Autodesk Fusion 360 part; units mm, degrees
(part 12 of 13)
  line L9839 (147.471, -118.112) -> (150.319, -115.264)
  line L9840 (149.69, -95.2494) -> (149.801, -95.1926)
  line L9841 (150.319, -98.5784) -> (149.809, -98.0678)
  line L9842 (149.787, -98.039) -> (149.781, -98.0089)
  line L9843 (149.525, -95.573) -> (149.544, -95.4494)
  line L9844 (139.992, -121.691) -> (139.992, -121.713)
  line L9845 (149.544, -95.6966) -> (149.525, -95.573)
  line L9846 (140.035, -118.135) -> (140.038, -118.132)
  line L9847 (137.265, -122.205) -> (137.136, -122.328)
  line L9848 (151.272, -97.8621) -> (151.28, -97.8916)
  line L9849 (151.002, -97.4818) -> (150.975, -97.5348)
  line L9850 (149.772, -95.9386) -> (149.69, -95.8966)
  line L9851 (149.801, -95.1926) -> (149.925, -95.173)
  line L9852 (151.022, -97.3582) -> (151.002, -97.4818)
  line L9853 (149.69, -95.8966) -> (149.601, -95.8081)
  line L9854 (151.265, -97.832) -> (151.272, -97.8621)
  line L9855 (149.792, -98.0469) -> (149.791, -98.0442)
  line L9856 (147.84, -118.96) -> (147.822, -118.974)
  line L9857 (147.752, -118.997) -> (142.062, -118.997)
  line L9858 (151.261, -97.8268) -> (151.265, -97.832)
  line L9859 (149.772, -97.9794) -> (149.772, -95.9387)
  line L9860 (149.781, -98.0089) -> (149.772, -97.9794)
  line L9861 (151.278, -115.495) -> (151.276, -115.498)
  line L9862 (140.017, -118.149) -> (140.035, -118.135)
  line L9863 (139.375, -120.912) -> (139.543, -120.972)
  line L9864 (139.967, -121.89) -> (139.904, -122.056)
  line L9865 (151.244, -115.557) -> (147.84, -118.96)
  line L9866 (139.353, -122.474) -> (139.175, -122.49)
  line L9867 (139.992, -121.713) -> (139.967, -121.89)
  line L9868 (150.387, -97.6818) -> (150.298, -97.5933)
  line L9869 (150.622, -97.7582) -> (150.498, -97.7386)
  line L9870 (138.409, -121.857) -> (138.392, -121.679)
  line L9871 (151.275, -115.504) -> (151.259, -115.53)
  line L9872 (147.817, -118.978) -> (147.811, -118.982)
  line L9873 (142.011, -118.747) -> (147.7, -118.747)
  line L9874 (138.466, -122.026) -> (138.409, -121.857)
  line L9875 (138.682, -122.307) -> (138.558, -122.179)
  line L9876 (150.746, -97.7386) -> (150.622, -97.7582)
  line L9877 (141.981, -118.756) -> (142.011, -118.747)
  line L9878 (138.414, -121.502) -> (138.475, -121.335)
  line L9879 (147.7, -118.747) -> (151.03, -115.417)
  line L9880 (147.811, -118.982) -> (147.781, -118.988)
  line L9881 (139.676, -122.328) -> (139.522, -122.419)
  line L9882 (150.242, -97.2346) -> (150.298, -97.1231)
  line L9883 (139.904, -122.056) -> (139.805, -122.205)
  line L9884 (151.276, -115.498) -> (151.275, -115.504)
  line L9885 (147.822, -118.974) -> (147.819, -118.977)
  line L9886 (147.781, -118.988) -> (147.752, -118.997)
  line L9887 (151.28, -97.8916) -> (151.28, -115.468)
  line L9888 (138.831, -122.405) -> (138.682, -122.307)
  line L9889 (147.819, -118.977) -> (147.817, -118.978)
  line L9890 (138.475, -121.335) -> (138.572, -121.185)
  line L9891 (139.913, -121.345) -> (139.972, -121.513)
  line L9892 (141.946, -118.766) -> (141.951, -118.762)
  line L9893 (150.799, -97.7116) -> (150.746, -97.7386)
  line L9894 (138.998, -122.467) -> (138.831, -122.405)
  line L9895 (139.543, -120.972) -> (139.66, -121.046)
  line L9896 (141.922, -118.784) -> (141.94, -118.77)
  line L9897 (151.28, -115.468) -> (151.277, -115.49)
  line L9898 (138.572, -121.185) -> (138.699, -121.06)
  line L9899 (139.522, -122.419) -> (139.353, -122.474)
  line L9900 (139.805, -122.205) -> (139.676, -122.328)
  line L9901 (139.175, -122.49) -> (138.998, -122.467)
  line L9902 (150.298, -97.5933) -> (150.242, -97.4818)
  line L9903 (141.94, -118.77) -> (141.943, -118.767)
  line L9904 (141.943, -118.767) -> (141.946, -118.766)
  line L9905 (150.242, -97.4818) -> (150.222, -97.3582)
  line L9906 (139.02, -120.909) -> (139.198, -120.891)
  line L9907 (150.498, -97.7386) -> (150.387, -97.6818)
  line L9908 (138.558, -122.179) -> (138.466, -122.026)
  line L9909 (151.03, -97.9434) -> (150.799, -97.7116)
  line L9910 (150.222, -97.3582) -> (150.242, -97.2346)
  line L9911 (118.089, -121.857) -> (118.072, -121.679)
  line L9912 (140.954, -121.502) -> (141.015, -121.335)
  line L9913 (119.356, -122.328) -> (119.202, -122.419)
  line L9914 (119.499, -121.194) -> (119.593, -121.345)
  line L9915 (138.392, -121.679) -> (138.414, -121.502)
  line L9916 (141.015, -121.335) -> (141.112, -121.185)
  line L9917 (142.512, -121.513) -> (142.532, -121.691)
  line L9918 (141.893, -122.474) -> (141.715, -122.49)
  line L9919 (151.03, -115.417) -> (151.03, -97.9434)
  line L9920 (141.371, -122.405) -> (141.222, -122.307)
  line L9921 (141.112, -121.185) -> (141.239, -121.06)
  line L9922 (140.949, -121.857) -> (140.932, -121.679)
  line L9923 (138.699, -121.06) -> (138.851, -120.967)
  line L9924 (139.66, -121.046) -> (141.922, -118.784)
  line L9925 (138.851, -120.967) -> (139.02, -120.909)
  line L9926 (139.198, -120.891) -> (139.375, -120.912)
  line L9927 (142.444, -122.056) -> (142.345, -122.205)
  line L9928 (142.345, -122.205) -> (142.216, -122.328)
  line L9929 (142.216, -122.328) -> (142.062, -122.419)
  line L9930 (141.915, -120.912) -> (142.083, -120.972)
  line L9931 (142.359, -121.194) -> (142.453, -121.345)
  line L9932 (150.298, -97.1231) -> (150.387, -97.0346)
  line L9933 (142.532, -121.713) -> (142.507, -121.89)
  line L9934 (142.532, -121.691) -> (142.532, -121.713)
  line L9935 (141.006, -122.026) -> (140.949, -121.857)
  line L9936 (140.932, -121.679) -> (140.954, -121.502)
  line L9937 (142.233, -121.067) -> (142.359, -121.194)
  line L9938 (150.622, -96.9582) -> (150.746, -96.9778)
  line L9939 (142.507, -121.89) -> (142.444, -122.056)
  line L9940 (141.391, -120.967) -> (141.56, -120.909)
  line L9941 (141.239, -121.06) -> (141.391, -120.967)
  line L9942 (142.062, -122.419) -> (141.893, -122.474)
  line L9943 (141.222, -122.307) -> (141.098, -122.179)
  line L9944 (142.083, -120.972) -> (142.233, -121.067)
  line L9945 (141.715, -122.49) -> (141.538, -122.467)
  line L9946 (141.538, -122.467) -> (141.371, -122.405)
  line L9947 (141.56, -120.909) -> (141.738, -120.891)
  line L9948 (118.379, -121.06) -> (118.531, -120.967)
  line L9949 (141.098, -122.179) -> (141.006, -122.026)
  line L9950 (142.453, -121.345) -> (142.512, -121.513)
  line L9951 (150.498, -96.9778) -> (150.622, -96.9582)
  line L9952 (118.531, -120.967) -> (118.7, -120.909)
  line L9953 (150.387, -97.0346) -> (150.498, -96.9778)
  line L9954 (119.373, -121.067) -> (119.499, -121.194)
  line L9955 (118.072, -121.679) -> (118.094, -121.502)
  line L9956 (131.594, -113.92) -> (131.706, -113.976)
  line L9957 (141.951, -118.762) -> (141.981, -118.756)
  line L9958 (119.652, -121.513) -> (119.672, -121.691)
  line L9959 (118.7, -120.909) -> (118.878, -120.891)
  line L9960 (122.124, -122.056) -> (122.025, -122.205)
  line L9961 (118.094, -121.502) -> (118.155, -121.335)
  line L9962 (121.537, -118.086) -> (121.537, -120.905)
  line L9963 (129.984, -115.963) -> (129.966, -115.977)
  line L9964 (119.672, -121.691) -> (119.672, -121.713)
  line L9965 (118.238, -122.179) -> (118.146, -122.026)
  line L9966 (122.025, -122.205) -> (121.896, -122.328)
  line L9967 (131.851, -114.176) -> (131.87, -114.3)
  line L9968 (122.212, -121.691) -> (122.212, -121.713)
  line L9969 (131.47, -114.7) -> (131.347, -114.68)
  line L9970 (131.706, -113.976) -> (131.794, -114.065)
  line L9971 (118.252, -121.185) -> (118.379, -121.06)
  line L9972 (121.763, -120.972) -> (121.913, -121.067)
  line L9973 (129.963, -115.98) -> (129.96, -115.981)
  line L9974 (118.146, -122.026) -> (118.089, -121.857)
  line L9975 (119.223, -120.972) -> (119.373, -121.067)
  line L9976 (122.192, -121.513) -> (122.212, -121.691)
  line L9977 (141.738, -120.891) -> (141.915, -120.912)
  line L9978 (129.955, -115.985) -> (129.925, -115.991)
  line L9979 (131.794, -114.065) -> (131.851, -114.176)
  line L9980 (122.039, -121.194) -> (122.133, -121.345)
  line L9981 (118.362, -122.307) -> (118.238, -122.179)
  line L9982 (119.647, -121.89) -> (119.584, -122.056)
  line L9983 (118.878, -120.891) -> (119.055, -120.912)
  line L9984 (119.672, -121.713) -> (119.647, -121.89)
  line L9985 (119.584, -122.056) -> (119.485, -122.205)
  line L9986 (118.855, -122.49) -> (118.678, -122.467)
  line L9987 (121.595, -120.912) -> (121.763, -120.972)
  line L9988 (118.155, -121.335) -> (118.252, -121.185)
  line L9989 (131.794, -114.535) -> (131.706, -114.624)
  line L9990 (119.202, -122.419) -> (119.033, -122.474)
  line L9991 (119.033, -122.474) -> (118.855, -122.49)
  line L9992 (118.678, -122.467) -> (118.511, -122.405)
  line L9993 (129.896, -116) -> (123.623, -116)
  line L9994 (121.896, -122.328) -> (121.742, -122.419)
  line L9995 (121.913, -121.067) -> (122.039, -121.194)
  line L9996 (122.133, -121.345) -> (122.192, -121.513)
  line L9997 (129.96, -115.981) -> (129.955, -115.985)
  line L9998 (123.623, -116) -> (121.537, -118.086)
  line L9999 (129.925, -115.991) -> (129.896, -116)
  line L10000 (131.87, -114.3) -> (131.851, -114.424)
  line L10001 (131.347, -114.68) -> (131.294, -114.653)
  line L10002 (119.593, -121.345) -> (119.652, -121.513)
  line L10003 (119.485, -122.205) -> (119.356, -122.328)
  line L10004 (118.511, -122.405) -> (118.362, -122.307)
  line L10005 (119.055, -120.912) -> (119.223, -120.972)
  line L10006 (122.187, -121.89) -> (122.124, -122.056)
  line L10007 (119.593, -116.06) -> (119.619, -116.076)
  line L10008 (121.537, -120.905) -> (121.595, -120.912)
  line L10009 (122.212, -121.713) -> (122.187, -121.89)
  line L10010 (131.594, -114.68) -> (131.47, -114.7)
  line L10011 (114.979, -115.856) -> (115.091, -115.799)
  line L10012 (120.686, -122.026) -> (120.629, -121.857)
  line L10013 (115.214, -116.58) -> (115.091, -116.56)
  line L10014 (121.287, -120.904) -> (121.287, -118.086)
  line L10015 (114.979, -116.503) -> (114.891, -116.415)
  line L10016 (115.338, -116.56) -> (115.214, -116.58)
  line L10017 (121.573, -122.474) -> (121.395, -122.49)
  line L10018 (115.091, -116.56) -> (114.979, -116.503)
  line L10019 (121.395, -122.49) -> (121.218, -122.467)
  line L10020 (119.58, -116.058) -> (119.584, -116.057)
  line L10021 (115.091, -115.799) -> (115.214, -115.78)
  line L10022 (131.47, -113.9) -> (131.594, -113.92)
  line L10023 (120.902, -122.307) -> (120.778, -122.179)
  line L10024 (116.515, -120.912) -> (116.683, -120.972)
  line L10025 (119.646, -116.091) -> (121.412, -117.857)
  line L10026 (120.792, -121.185) -> (120.919, -121.06)
  line L10027 (131.851, -114.424) -> (131.794, -114.535)
  line L10028 (131.706, -114.624) -> (131.594, -114.68)
  line L10029 (129.966, -115.977) -> (129.963, -115.98)
  line L10030 (120.612, -121.679) -> (120.634, -121.502)
  line L10031 (115.538, -116.415) -> (115.45, -116.503)
  line L10032 (121.051, -122.405) -> (120.902, -122.307)
  line L10033 (131.294, -114.653) -> (129.984, -115.963)
  line L10034 (120.634, -121.502) -> (120.695, -121.335)
  line L10035 (120.629, -121.857) -> (120.612, -121.679)
  line L10036 (120.695, -121.335) -> (120.792, -121.185)
  line L10037 (115.594, -116.305) -> (115.538, -116.415)
  line L10038 (114.891, -115.944) -> (114.979, -115.856)
  line L10039 (120.919, -121.06) -> (121.071, -120.967)
  line L10040 (119.506, -116.305) -> (115.594, -116.305)
  line L10041 (121.287, -118.086) -> (119.506, -116.305)
  line L10042 (114.834, -116.056) -> (114.891, -115.944)
  line L10043 (114.814, -116.18) -> (114.834, -116.056)
  line L10044 (114.891, -116.415) -> (114.834, -116.303)
  line L10045 (121.071, -120.967) -> (121.24, -120.909)
  line L10046 (121.742, -122.419) -> (121.573, -122.474)
  line L10047 (114.834, -116.303) -> (114.814, -116.18)
  line L10048 (131.347, -113.92) -> (131.47, -113.9)
  line L10049 (115.45, -115.856) -> (115.538, -115.944)
  line L10050 (121.24, -120.909) -> (121.287, -120.904)
  line L10051 (131.07, -114.3) -> (131.09, -114.176)
  line L10052 (120.778, -122.179) -> (120.686, -122.026)
  line L10053 (121.218, -122.467) -> (121.051, -122.405)
  line L10054 (115.45, -116.503) -> (115.338, -116.56)
  line L10055 (115.338, -115.799) -> (115.45, -115.856)
  line L10056 (119.619, -116.076) -> (119.646, -116.091)
  line L10057 (129.844, -115.75) -> (131.117, -114.477)
  line L10058 (115.712, -121.185) -> (115.839, -121.06)
  line L10059 (121.412, -117.857) -> (123.483, -115.786)
  line L10060 (116.959, -121.194) -> (117.053, -121.345)
  line L10061 (123.5, -115.773) -> (123.503, -115.77)
  line L10062 (116.138, -122.467) -> (115.971, -122.405)
  line L10063 (124.673, -121.345) -> (124.732, -121.513)
  line L10064 (123.541, -115.758) -> (123.571, -115.75)
  line L10065 (115.532, -121.679) -> (115.554, -121.502)
  line L10066 (115.698, -122.179) -> (115.606, -122.026)
  line L10067 (116.683, -120.972) -> (116.833, -121.067)
  line L10068 (119.558, -116.055) -> (119.58, -116.058)
  line L10069 (115.538, -115.944) -> (115.594, -116.055)
  line L10070 (123.503, -115.77) -> (123.506, -115.769)
  line L10071 (115.606, -122.026) -> (115.549, -121.857)
  line L10072 (123.511, -115.765) -> (123.541, -115.758)
  line L10073 (116.816, -122.328) -> (116.662, -122.419)
  line L10074 (115.971, -122.405) -> (115.822, -122.307)
  line L10075 (116.662, -122.419) -> (116.493, -122.474)
  line L10076 (115.991, -120.967) -> (116.16, -120.909)
  line L10077 (123.571, -115.75) -> (129.844, -115.75)
  line L10078 (115.214, -115.78) -> (115.338, -115.799)
  line L10079 (117.132, -121.691) -> (117.132, -121.713)
  line L10080 (119.587, -116.059) -> (119.593, -116.06)
  line L10081 (131.117, -114.477) -> (131.09, -114.424)
  line L10082 (131.235, -113.976) -> (131.347, -113.92)
  line L10083 (116.945, -122.205) -> (116.816, -122.328)
  line L10084 (123.506, -115.769) -> (123.511, -115.765)
  line L10085 (115.594, -116.055) -> (119.558, -116.055)
  line L10086 (116.338, -120.891) -> (116.515, -120.912)
  line L10087 (115.822, -122.307) -> (115.698, -122.179)
  line L10088 (116.16, -120.909) -> (116.338, -120.891)
  line L10089 (117.107, -121.89) -> (117.044, -122.056)
  line L10090 (116.493, -122.474) -> (116.315, -122.49)
  line L10091 (131.09, -114.424) -> (131.07, -114.3)
  line L10092 (115.554, -121.502) -> (115.615, -121.335)
  line L10093 (131.09, -114.176) -> (131.147, -114.065)
  line L10094 (115.615, -121.335) -> (115.712, -121.185)
  line L10095 (115.839, -121.06) -> (115.991, -120.967)
  line L10096 (131.147, -114.065) -> (131.235, -113.976)
  line L10097 (115.549, -121.857) -> (115.532, -121.679)
  line L10098 (117.044, -122.056) -> (116.945, -122.205)
  line L10099 (123.483, -115.786) -> (123.5, -115.773)
  line L10100 (119.584, -116.057) -> (119.587, -116.059)
  line L10101 (124.135, -120.912) -> (124.303, -120.972)
  line L10102 (124.453, -121.067) -> (124.579, -121.194)
  line L10103 (117.112, -121.513) -> (117.132, -121.691)
  line L10104 (124.565, -122.205) -> (124.436, -122.328)
  line L10105 (148.706, -104.986) -> (148.715, -105.016)
  line L10106 (146.816, -116.702) -> (146.787, -116.711)
  line L10107 (124.303, -120.972) -> (124.453, -121.067)
  line L10108 (123.152, -121.679) -> (123.174, -121.502)
  line L10109 (146.679, -102.546) -> (146.768, -102.635)
  line L10110 (124.113, -122.474) -> (123.935, -122.49)
  line L10111 (123.169, -121.857) -> (123.152, -121.679)
  line L10112 (146.568, -102.49) -> (146.679, -102.546)
  line L10113 (123.935, -122.49) -> (123.758, -122.467)
  line L10114 (123.591, -122.405) -> (123.442, -122.307)
  line L10115 (123.442, -122.307) -> (123.318, -122.179)
  line L10116 (124.732, -121.513) -> (124.752, -121.691)
  line L10117 (146.798, -103.047) -> (148.678, -104.927)
  line L10118 (123.78, -120.909) -> (123.958, -120.891)
  line L10119 (148.71, -114.818) -> (148.693, -114.844)
  line L10120 (146.857, -116.688) -> (146.854, -116.691)
  line L10121 (146.825, -102.746) -> (146.844, -102.87)
  line L10122 (123.235, -121.335) -> (123.332, -121.185)
  line L10123 (148.712, -114.809) -> (148.711, -114.812)
  line L10124 (124.752, -121.713) -> (124.727, -121.89)
  line L10125 (123.332, -121.185) -> (123.459, -121.06)
  line L10126 (123.758, -122.467) -> (123.591, -122.405)
  line L10127 (124.436, -122.328) -> (124.282, -122.419)
  line L10128 (117.053, -121.345) -> (117.112, -121.513)
  line L10129 (126.653, -122.474) -> (126.475, -122.49)
  line L10130 (124.579, -121.194) -> (124.673, -121.345)
  line L10131 (146.825, -102.994) -> (146.798, -103.047)
  line L10132 (123.226, -122.026) -> (123.169, -121.857)
  line L10133 (146.844, -102.87) -> (146.825, -102.994)
  line L10134 (124.664, -122.056) -> (124.565, -122.205)
  line L10135 (148.715, -105.016) -> (148.715, -114.783)
  line L10136 (116.315, -122.49) -> (116.138, -122.467)
  line L10137 (123.318, -122.179) -> (123.226, -122.026)
  line L10138 (123.958, -120.891) -> (124.135, -120.912)
  line L10139 (127.272, -121.513) -> (127.292, -121.691)
  line L10140 (148.678, -104.927) -> (148.692, -104.945)
  line L10141 (124.727, -121.89) -> (124.664, -122.056)
  line L10142 (123.611, -120.967) -> (123.78, -120.909)
  line L10143 (146.768, -102.635) -> (146.825, -102.746)
  line L10144 (124.752, -121.691) -> (124.752, -121.713)
  line L10145 (123.459, -121.06) -> (123.611, -120.967)
  line L10146 (148.692, -104.945) -> (148.695, -104.948)
  line L10147 (116.833, -121.067) -> (116.959, -121.194)
  line L10148 (123.174, -121.502) -> (123.235, -121.335)
  line L10149 (117.132, -121.713) -> (117.107, -121.89)
  line L10150 (124.282, -122.419) -> (124.113, -122.474)
  line L10151 (125.709, -121.857) -> (125.692, -121.679)
  line L10152 (148.693, -114.844) -> (148.678, -114.871)
  line L10153 (125.692, -121.679) -> (125.714, -121.502)
  line L10154 (126.822, -122.419) -> (126.653, -122.474)
  line L10155 (126.675, -120.912) -> (126.843, -120.972)
  line L10156 (126.298, -122.467) -> (126.131, -122.405)
  line L10157 (126.475, -122.49) -> (126.298, -122.467)
  line L10158 (131.567, -116.47) -> (131.597, -116.461)
  line L10159 (131.648, -116.711) -> (127.137, -121.222)
  line L10160 (146.568, -103.25) -> (146.444, -103.27)
  line L10161 (127.204, -122.056) -> (127.105, -122.205)
  line L10162 (126.843, -120.972) -> (126.96, -121.046)
  line L10163 (125.872, -121.185) -> (125.999, -121.06)
  line L10164 (127.213, -121.345) -> (127.272, -121.513)
  line L10165 (146.444, -103.27) -> (146.321, -103.25)
  line L10166 (126.32, -120.909) -> (126.498, -120.891)
  line L10167 (148.715, -114.783) -> (148.712, -114.805)
  line L10168 (125.858, -122.179) -> (125.766, -122.026)
  line L10169 (126.976, -122.328) -> (126.822, -122.419)
  line L10170 (148.711, -114.812) -> (148.71, -114.818)
  line L10171 (127.292, -121.691) -> (127.292, -121.713)
  line L10172 (148.7, -104.956) -> (148.706, -104.986)
  line L10173 (148.695, -104.948) -> (148.696, -104.951)
  line L10174 (127.292, -121.713) -> (127.267, -121.89)
  line L10175 (146.851, -116.692) -> (146.846, -116.696)
  line L10176 (148.678, -114.871) -> (146.875, -116.674)
  line L10177 (127.137, -121.222) -> (127.213, -121.345)
  line L10178 (127.267, -121.89) -> (127.204, -122.056)
  line L10179 (126.498, -120.891) -> (126.675, -120.912)
  line L10180 (146.854, -116.691) -> (146.851, -116.692)
  line L10181 (148.696, -104.951) -> (148.7, -104.956)
  line L10182 (148.712, -114.805) -> (148.712, -114.809)
  line L10183 (146.875, -116.674) -> (146.857, -116.688)
  line L10184 (127.105, -122.205) -> (126.976, -122.328)
  line L10185 (146.787, -116.711) -> (131.648, -116.711)
  line L10186 (146.735, -116.461) -> (148.465, -114.731)
  line L10187 (125.714, -121.502) -> (125.775, -121.335)
  line L10188 (125.982, -122.307) -> (125.858, -122.179)
  line L10189 (131.532, -116.48) -> (131.537, -116.476)
  line L10190 (131.526, -116.484) -> (131.529, -116.481)
  line L10191 (146.621, -103.223) -> (146.568, -103.25)
  line L10192 (125.766, -122.026) -> (125.709, -121.857)
  line L10193 (126.131, -122.405) -> (125.982, -122.307)
  line L10194 (126.151, -120.967) -> (126.32, -120.909)
  line L10195 (148.465, -105.067) -> (146.621, -103.223)
  line L10196 (146.846, -116.696) -> (146.816, -116.702)
  line L10197 (131.537, -116.476) -> (131.567, -116.47)
  line L10198 (125.775, -121.335) -> (125.872, -121.185)
  line L10199 (128.315, -121.335) -> (128.412, -121.185)
  line L10200 (128.522, -122.307) -> (128.398, -122.179)
  line L10201 (129.832, -121.713) -> (129.807, -121.89)
  line L10202 (104.265, -111.959) -> (104.184, -112.013)
  line L10203 (128.838, -122.467) -> (128.671, -122.405)
  line L10204 (129.383, -120.972) -> (129.533, -121.067)
  line L10205 (104.184, -112.013) -> (104.088, -112.032)
  line L10206 (101.788, -109.313) -> (101.804, -109.325)
  line L10207 (129.812, -121.513) -> (129.832, -121.691)
  line L10208 (104.088, -112.032) -> (102.873, -112.032)
  line L10209 (146.121, -102.635) -> (146.209, -102.546)
  line L10210 (126.96, -121.046) -> (131.508, -116.498)
  line L10211 (129.215, -120.912) -> (129.383, -120.972)
  line L10212 (128.398, -122.179) -> (128.306, -122.026)
  line L10213 (128.306, -122.026) -> (128.249, -121.857)
  line L10214 (128.254, -121.502) -> (128.315, -121.335)
  line L10215 (129.807, -121.89) -> (129.744, -122.056)
  line L10216 (129.659, -121.194) -> (129.753, -121.345)
  line L10217 (125.999, -121.06) -> (126.151, -120.967)
  line L10218 (146.044, -102.87) -> (146.064, -102.746)
  line L10219 (146.209, -103.194) -> (146.121, -103.105)
  line L10220 (146.121, -103.105) -> (146.064, -102.994)
  line L10221 (148.465, -114.731) -> (148.465, -105.067)
  line L10222 (128.232, -121.679) -> (128.254, -121.502)
  line L10223 (129.015, -122.49) -> (128.838, -122.467)
  line L10224 (146.321, -102.49) -> (146.444, -102.47)
  line L10225 (131.508, -116.498) -> (131.526, -116.484)
  line L10226 (131.597, -116.461) -> (146.735, -116.461)
  line L10227 (129.753, -121.345) -> (129.812, -121.513)
  line L10228 (146.444, -102.47) -> (146.568, -102.49)
  line L10229 (128.671, -122.405) -> (128.522, -122.307)
  line L10230 (129.362, -122.419) -> (129.193, -122.474)
  line L10231 (101.604, -109.259) -> (101.655, -109.263)
  line L10232 (129.516, -122.328) -> (129.362, -122.419)
  line L10233 (129.645, -122.205) -> (129.516, -122.328)
  line L10234 (129.744, -122.056) -> (129.645, -122.205)
  line L10235 (146.321, -103.25) -> (146.209, -103.194)
  line L10236 (146.209, -102.546) -> (146.321, -102.49)
  line L10237 (146.064, -102.994) -> (146.044, -102.87)
  line L10238 (131.529, -116.481) -> (131.532, -116.48)
  line L10239 (129.832, -121.691) -> (129.832, -121.713)
  line L10240 (129.193, -122.474) -> (129.015, -122.49)
  line L10241 (146.064, -102.746) -> (146.121, -102.635)
  line L10242 (129.533, -121.067) -> (129.659, -121.194)
  line L10243 (101.74, -109.295) -> (101.788, -109.313)
  line L10244 (104.319, -111.878) -> (104.265, -111.959)
  line L10245 (104.338, -111.782) -> (104.319, -111.878)
  line L10246 (128.249, -121.857) -> (128.232, -121.679)
  line L10247 (101.804, -109.325) -> (101.822, -109.334)
  line L10248 (103.41, -110.907) -> (104.088, -110.907)
  line L10249 (100.614, -112.96) -> (100.636, -112.914)
  line L10250 (100.366, -122.026) -> (100.309, -121.857)
  line L10251 (101.694, -109.273) -> (101.74, -109.295)
  line L10252 (101.892, -121.713) -> (101.867, -121.89)
  line L10253 (102.873, -112.032) -> (101.592, -113.313)
  line L10254 (101.253, -122.474) -> (101.075, -122.49)
  line L10255 (101.813, -121.345) -> (101.872, -121.513)
  line L10256 (101.075, -122.49) -> (100.898, -122.467)
  line L10257 (100.731, -122.405) -> (100.582, -122.307)
  line L10258 (101.576, -122.328) -> (101.422, -122.419)
  line L10259 (100.309, -121.857) -> (100.292, -121.679)
  line L10260 (101.593, -121.067) -> (101.719, -121.194)
  line L10261 (104.338, -111.157) -> (104.338, -111.782)
  line L10262 (101.892, -121.691) -> (101.892, -121.713)
  line L10263 (101.655, -109.263) -> (101.674, -109.27)
  line L10264 (128.539, -121.06) -> (128.691, -120.967)
  line L10265 (101.674, -109.27) -> (101.694, -109.273)
  line L10266 (101.822, -109.334) -> (101.86, -109.367)
  line L10267 (129.038, -120.891) -> (129.215, -120.912)
  line L10268 (104.088, -110.907) -> (104.184, -110.926)
  line L10269 (104.265, -110.981) -> (104.319, -111.062)
  line L10270 (101.86, -109.367) -> (101.901, -109.398)
  line L10271 (101.547, -109.252) -> (101.554, -109.252)
  line L10272 (100.472, -121.185) -> (100.592, -121.068)
  line L10273 (101.804, -122.056) -> (101.705, -122.205)
  line L10274 (100.611, -112.98) -> (100.614, -112.96)
  line L10275 (101.422, -122.419) -> (101.253, -122.474)
  line L10276 (100.592, -121.068) -> (100.592, -113.106)
  line L10277 (100.604, -112.999) -> (100.611, -112.98)
  line L10278 (128.412, -121.185) -> (128.539, -121.06)
  line L10279 (128.691, -120.967) -> (128.86, -120.909)
  line L10280 (101.872, -121.513) -> (101.892, -121.691)
  line L10281 (128.86, -120.909) -> (129.038, -120.891)
  line L10282 (101.901, -109.398) -> (103.41, -110.907)
  line L10283 (101.719, -121.194) -> (101.813, -121.345)
  line L10284 (100.375, -121.335) -> (100.472, -121.185)
  line L10285 (104.319, -111.062) -> (104.338, -111.157)
  line L10286 (101.554, -109.252) -> (101.604, -109.259)
  line L10287 (100.636, -112.914) -> (100.653, -112.866)
  line L10288 (101.592, -121.066) -> (101.593, -121.067)
  line L10289 (101.592, -113.313) -> (101.592, -121.066)
  line L10290 (101.073, -109.252) -> (101.547, -109.252)
  line L10291 (100.592, -113.106) -> (100.592, -113.1)
  line L10292 (100.314, -121.502) -> (100.375, -121.335)
  line L10293 (104.184, -110.926) -> (104.265, -110.981)
  line L10294 (100.6, -113.05) -> (100.604, -112.999)
  line L10295 (100.653, -112.866) -> (100.666, -112.85)
  line L10296 (100.708, -112.793) -> (100.738, -112.753)
  line L10297 (101.867, -121.89) -> (101.804, -122.056)
  line L10298 (100.898, -122.467) -> (100.731, -122.405)
  line L10299 (101.521, -111.97) -> (101.073, -111.97)
  line L10300 (100.738, -112.753) -> (101.521, -111.97)
  line L10301 (115.569, -112.441) -> (115.566, -112.44)
  line L10302 (112.508, -111.86) -> (112.508, -112.189)
  line L10303 (115.56, -112.439) -> (115.534, -112.422)
  line L10304 (116.587, -110.754) -> (116.592, -110.761)
  line L10305 (116.593, -111.918) -> (116.592, -111.926)
  line L10306 (101.073, -110.97) -> (102.059, -110.97)
  line L10307 (100.582, -122.307) -> (100.458, -122.179)
  line L10308 (116.515, -112.026) -> (116.515, -112.03)
  line L10309 (114.511, -112.485) -> (114.511, -112.335)
  line L10310 (101.073, -111.97) -> (101.073, -112.002)
  line L10311 (116.078, -112.444) -> (115.595, -112.444)
  line L10312 (101.073, -112.002) -> (96.4732, -112.002)
  line L10313 (96.4732, -112.002) -> (96.4732, -110.902)
  line L10314 (101.073, -110.902) -> (101.073, -110.97)
  line L10315 (100.674, -112.832) -> (100.708, -112.793)
  line L10316 (116.581, -111.937) -> (116.573, -111.938)
  line L10317 (116.513, -112.039) -> (116.496, -112.065)
  line L10318 (116.518, -111.938) -> (116.518, -112.004)
  line L10319 (102.059, -110.97) -> (101.34, -110.252)
  line L10320 (116.108, -112.435) -> (116.078, -112.444)
  line L10321 (116.573, -111.938) -> (116.518, -111.938)
  line L10322 (100.666, -112.85) -> (100.674, -112.832)
  line L10323 (116.593, -110.768) -> (116.593, -111.918)
  line L10324 (100.458, -122.179) -> (100.366, -122.026)
  line L10325 (101.073, -110.252) -> (101.073, -110.302)
  line L10326 (96.4732, -110.902) -> (101.073, -110.902)
  line L10327 (96.4732, -110.302) -> (96.4732, -109.202)
  line L10328 (111.247, -112.439) -> (110.927, -112.759)
  line L10329 (116.514, -112.033) -> (116.513, -112.039)
  line L10330 (116.592, -110.761) -> (116.593, -110.768)
  line L10331 (101.073, -110.302) -> (96.4732, -110.302)
  line L10332 (96.4732, -109.202) -> (101.073, -109.202)
  line L10333 (100.292, -121.679) -> (100.314, -121.502)
  line L10334 (101.705, -122.205) -> (101.576, -122.328)
  line L10335 (101.073, -109.202) -> (101.073, -109.252)
  line L10336 (116.592, -111.926) -> (116.587, -111.932)
  line L10337 (116.581, -110.75) -> (116.587, -110.754)
  line L10338 (100.592, -113.1) -> (100.6, -113.05)
  line L10339 (116.518, -112.004) -> (116.515, -112.026)
  line L10340 (116.515, -112.03) -> (116.514, -112.033)
  line L10341 (116.587, -111.932) -> (116.581, -111.937)
  line L10342 (101.34, -110.252) -> (101.073, -110.252)
  line L10343 (130.364, -112.199) -> (130.345, -112.295)
  line L10344 (130.114, -111.324) -> (130.21, -111.343)
  line L10345 (128.85, -114.359) -> (130.127, -113.082)
  line L10346 (114.511, -112.335) -> (114.211, -112.335)
  line L10347 (115.566, -112.44) -> (115.56, -112.439)
  line L10348 (112.508, -112.189) -> (112.489, -112.284)
  line L10349 (113.211, -111.86) -> (112.508, -111.86)
  line L10350 (112.435, -112.366) -> (112.354, -112.42)
  line L10351 (110.927, -112.759) -> (112.526, -114.359)
  line L10352 (128.687, -111.398) -> (128.769, -111.343)
  line L10353 (116.149, -112.421) -> (116.146, -112.424)
  line L10354 (130.127, -113.082) -> (129.494, -112.449)
  line L10355 (112.258, -112.439) -> (111.247, -112.439)
  line L10356 (114.211, -112.335) -> (114.211, -112.485)
  line L10357 (112.526, -114.359) -> (128.85, -114.359)
  line L10358 (128.864, -111.324) -> (130.114, -111.324)
  line L10359 (128.769, -112.43) -> (128.687, -112.376)
  line L10360 (128.687, -112.376) -> (128.633, -112.295)
  line L10361 (130.291, -111.398) -> (130.345, -111.479)
  line L10362 (128.864, -112.449) -> (128.769, -112.43)
  line L10363 (128.633, -112.295) -> (128.614, -112.199)
  line L10364 (116.496, -112.065) -> (116.482, -112.092)
  line L10365 (112.489, -112.284) -> (112.435, -112.366)
  line L10366 (130.799, -112.659) -> (130.938, -112.69)
  line L10367 (113.211, -112.485) -> (113.211, -111.86)
  line L10368 (115.534, -112.422) -> (115.511, -112.409)
  line L10369 (112.354, -112.42) -> (112.258, -112.439)
  line L10370 (116.143, -112.425) -> (116.138, -112.429)
  line L10371 (116.146, -112.424) -> (116.143, -112.425)
  line L10372 (130.21, -111.343) -> (130.291, -111.398)
  line L10373 (130.658, -112.667) -> (130.799, -112.659)
  line L10374 (116.138, -112.429) -> (116.108, -112.435)
  line L10375 (115.511, -112.485) -> (114.511, -112.485)
  line L10376 (115.595, -112.444) -> (115.573, -112.441)
  line L10377 (115.511, -112.409) -> (115.511, -112.485)
  line L10378 (128.614, -111.574) -> (128.633, -111.479)
  line L10379 (128.769, -111.343) -> (128.864, -111.324)
  line L10380 (130.345, -111.479) -> (130.364, -111.574)
  line L10381 (116.166, -112.407) -> (116.149, -112.421)
  line L10382 (130.345, -112.295) -> (130.291, -112.376)
  line L10383 (116.482, -112.092) -> (116.166, -112.407)
  line L10384 (128.614, -112.199) -> (128.614, -111.574)
  line L10385 (114.211, -112.485) -> (113.211, -112.485)
  line L10386 (129.494, -112.449) -> (128.864, -112.449)
  line L10387 (130.291, -112.376) -> (130.21, -112.43)
  line L10388 (115.573, -112.441) -> (115.569, -112.441)
  line L10389 (129.847, -112.449) -> (130.304, -112.906)
  line L10390 (130.41, -112.799) -> (130.524, -112.716)
  line L10391 (134.376, -111.686) -> (134.376, -111.681)
  line L10392 (128.633, -111.479) -> (128.687, -111.398)
  line L10393 (134.309, -111.686) -> (134.376, -111.686)
  line L10394 (131.078, -112.199) -> (131.078, -111.574)
  line L10395 (131.328, -112.449) -> (131.232, -112.43)
  line L10396 (131.161, -112.86) -> (131.228, -112.984)
  line L10397 (131.151, -112.376) -> (131.097, -112.295)
  line L10398 (131.078, -111.574) -> (131.097, -111.479)
  line L10399 (133.876, -112.306) -> (133.876, -112.181)
  line L10400 (132.339, -112.449) -> (132.077, -112.449)
  line L10401 (131.328, -111.324) -> (132.578, -111.324)
  line L10402 (134.161, -113.132) -> (134.043, -113.054)
  line L10403 (130.524, -112.716) -> (130.658, -112.667)
  line L10404 (131.773, -112.449) -> (131.328, -112.449)
  line L10405 (132.755, -111.398) -> (132.809, -111.479)
  line L10406 (130.21, -112.43) -> (130.114, -112.449)
  line L10407 (130.364, -111.574) -> (130.364, -112.199)
  line L10408 (130.304, -112.906) -> (130.406, -112.803)
  line L10409 (133.876, -112.175) -> (133.898, -112.035)
  line L10410 (132.828, -111.574) -> (132.828, -112.199)
  line L10411 (133.876, -112.181) -> (133.877, -112.181)
  line L10412 (130.938, -112.69) -> (131.061, -112.759)
  line L10413 (131.232, -111.343) -> (131.328, -111.324)
  line L10414 (132.578, -111.324) -> (132.674, -111.343)
  line L10415 (131.23, -112.992) -> (131.773, -112.449)
  line L10416 (131.232, -112.43) -> (131.151, -112.376)
  line L10417 (132.674, -111.343) -> (132.755, -111.398)
  line L10418 (134.043, -113.054) -> (133.952, -112.945)
  line L10419 (132.809, -112.295) -> (132.802, -112.306)
  line L10420 (133.952, -112.945) -> (133.895, -112.815)
  line L10421 (131.097, -111.479) -> (131.151, -111.398)
  line L10422 (132.077, -112.449) -> (132.075, -112.468)
  line L10423 (132.809, -111.479) -> (132.828, -111.574)
  line L10424 (133.958, -111.906) -> (134.052, -111.8)
  line L10425 (130.114, -112.449) -> (129.847, -112.449)
  line L10426 (130.406, -112.803) -> (130.41, -112.799)
  line L10427 (134.172, -111.725) -> (134.309, -111.686)
  line L10428 (132.828, -112.199) -> (132.809, -112.295)
  line L10429 (131.228, -112.984) -> (131.23, -112.992)
  line L10430 (133.898, -112.035) -> (133.958, -111.906)
  line L10431 (132.802, -112.306) -> (133.876, -112.306)
  line L10432 (131.097, -112.295) -> (131.078, -112.199)
  line L10433 (131.061, -112.759) -> (131.161, -112.86)
  line L10434 (131.151, -111.398) -> (131.232, -111.343)
  line L10435 (134.052, -111.8) -> (134.172, -111.725)
  line L10436 (133.895, -112.815) -> (133.877, -112.681)
  line L10437 (132.47, -112.553) -> (132.468, -112.552)
  line L10438 (133.877, -112.181) -> (133.876, -112.175)
  line L10439 (132.462, -112.551) -> (132.436, -112.534)
  line L10440 (111.865, -122.205) -> (111.736, -122.328)
  line L10441 (129.178, -115.342) -> (129.159, -115.348)
  line L10442 (129.327, -115.28) -> (129.308, -115.288)
  line L10443 (133.876, -112.681) -> (133.876, -112.556)
  line L10444 (129.411, -115.212) -> (129.407, -115.217)
  line L10445 (131.113, -113.511) -> (129.411, -115.212)
  line L10446 (131.241, -113.282) -> (131.198, -113.397)
  line L10447 (131.312, -113.259) -> (131.309, -113.262)
  line L10448 (129.159, -115.348) -> (129.108, -115.352)
  line L10449 (111.736, -122.328) -> (111.582, -122.419)
  line L10450 (131.242, -113.282) -> (131.241, -113.282)
  line L10451 (129.057, -115.359) -> (112.526, -115.359)
  line L10452 (129.198, -115.339) -> (129.178, -115.342)
  line L10453 (132.075, -112.472) -> (132.074, -112.475)
  line L10454 (131.33, -113.245) -> (131.312, -113.259)
  line L10455 (132.074, -112.475) -> (132.073, -112.481)
  line L10456 (131.198, -113.397) -> (131.113, -113.511)
  line L10457 (112.052, -121.691) -> (112.052, -121.713)
  line L10458 (111.964, -122.056) -> (111.865, -122.205)
  line L10459 (111.973, -121.345) -> (112.032, -121.513)
  line L10460 (129.108, -115.352) -> (129.057, -115.359)
  line L10461 (133.877, -112.681) -> (133.876, -112.681)
  line L10462 (129.308, -115.288) -> (129.292, -115.3)
  line L10463 (129.407, -115.217) -> (129.365, -115.247)
  line L10464 (132.073, -112.481) -> (132.056, -112.507)
  line L10465 (132.468, -112.552) -> (132.462, -112.551)
  line L10466 (134.376, -113.181) -> (134.376, -113.176)
  line L10467 (134.376, -113.176) -> (134.296, -113.175)
  line L10468 (134.296, -113.175) -> (134.161, -113.132)
  line L10469 (134.876, -113.181) -> (134.376, -113.181)
  line L10470 (132.475, -112.553) -> (132.47, -112.553)
  line L10471 (132.056, -112.507) -> (132.041, -112.534)
  line L10472 (132.041, -112.534) -> (131.33, -113.245)
  line L10473 (111.93, -115.955) -> (111.93, -121.275)
  line L10474 (132.409, -112.519) -> (132.339, -112.449)
  line L10475 (131.309, -113.262) -> (131.307, -113.263)
  line L10476 (134.876, -111.681) -> (134.876, -113.181)
  line L10477 (132.075, -112.468) -> (132.075, -112.472)
  line L10478 (111.582, -122.419) -> (111.413, -122.474)
  line L10479 (112.032, -121.513) -> (112.052, -121.691)
  line L10480 (132.436, -112.534) -> (132.409, -112.519)
  line L10481 (131.301, -113.267) -> (131.271, -113.273)
  line L10482 (129.365, -115.247) -> (129.327, -115.28)
  line L10483 (133.876, -112.556) -> (132.497, -112.556)
  line L10484 (134.376, -111.681) -> (134.876, -111.681)
  line L10485 (132.497, -112.556) -> (132.475, -112.553)
  line L10486 (111.93, -121.275) -> (111.973, -121.345)
  line L10487 (110.354, -112.43) -> (110.496, -112.44)
  line L10488 (110.474, -121.502) -> (110.535, -121.335)
  line L10489 (110.93, -115.742) -> (110.938, -115.691)
  line L10490 (110.891, -122.405) -> (110.742, -122.307)
  line L10491 (111.003, -115.492) -> (111.012, -115.473)
  line L10492 (110.759, -121.06) -> (110.911, -120.967)
  line L10493 (111.058, -122.467) -> (110.891, -122.405)
  line L10494 (112.052, -121.713) -> (112.027, -121.89)
  line L10495 (110.618, -122.179) -> (110.526, -122.026)
  line L10496 (110.742, -122.307) -> (110.618, -122.179)
  line L10497 (110.941, -115.64) -> (110.949, -115.622)
  line L10498 (111.612, -114.859) -> (110.035, -113.282)
  line L10499 (110.035, -113.282) -> (110.031, -113.278)
  line L10500 (109.864, -112.42) -> (110.031, -112.586)
  line L10501 (110.629, -112.49) -> (110.742, -112.575)
  line L10502 (110.452, -121.679) -> (110.474, -121.502)
  line L10503 (109.947, -113.163) -> (109.899, -113.03)
  line L10504 (112.526, -115.359) -> (111.93, -115.955)
  line L10505 (111.012, -115.473) -> (111.046, -115.435)
  line L10506 (109.864, -112.42) -> (109.864, -112.42)
  line L10507 (112.027, -121.89) -> (111.964, -122.056)
  line L10508 (110.526, -122.026) -> (110.469, -121.857)
  line L10509 (129.292, -115.3) -> (129.244, -115.318)
  line L10510 (111.413, -122.474) -> (111.235, -122.49)
  line L10511 (110.031, -113.278) -> (109.947, -113.163)
  line L10512 (110.973, -115.555) -> (110.991, -115.508)
  line L10513 (110.938, -115.691) -> (110.941, -115.64)
  line L10514 (110.535, -121.335) -> (110.632, -121.185)
  line L10515 (129.244, -115.318) -> (129.198, -115.339)
  line L10516 (110.469, -121.857) -> (110.452, -121.679)
  line L10517 (110.949, -115.622) -> (110.952, -115.602)
  line L10518 (111.235, -122.49) -> (111.058, -122.467)
  line L10519 (111.076, -115.394) -> (111.612, -114.859)
  line L10520 (110.632, -121.185) -> (110.759, -121.06)
  line L10521 (131.307, -113.263) -> (131.301, -113.267)
  line L10522 (109.899, -113.03) -> (109.89, -112.888)
  line L10523 (110.93, -115.748) -> (110.93, -115.742)
  line L10524 (110.952, -115.602) -> (110.973, -115.555)
  line L10525 (110.991, -115.508) -> (111.003, -115.492)
  line L10526 (111.046, -115.435) -> (111.076, -115.394)
  line L10527 (110.93, -120.96) -> (110.93, -115.748)
  line L10528 (131.271, -113.273) -> (131.242, -113.282)
  line L10529 (109.906, -112.816) -> (109.53, -112.439)
  line L10530 (108.288, -112.284) -> (108.269, -112.189)
  line L10531 (109.864, -111.333) -> (109.946, -111.387)
  line L10532 (108.519, -111.314) -> (109.769, -111.314)
  line L10533 (110.911, -120.967) -> (110.93, -120.96)
  line L10534 (110, -111.468) -> (110.019, -111.564)
  line L10535 (110.496, -112.44) -> (110.629, -112.49)
  line L10536 (113.211, -110.985) -> (114.211, -110.985)
  line L10537 (110.777, -111.468) -> (110.831, -111.387)
  line L10538 (110.758, -111.564) -> (110.777, -111.468)
  line L10539 (109.769, -111.314) -> (109.864, -111.333)
  line L10540 (116.268, -111.952) -> (116.268, -111.938)
  line L10541 (115.647, -112.194) -> (116.026, -112.194)
  line L10542 (116.193, -111.918) -> (116.193, -110.768)
  line L10543 (115.511, -112.058) -> (115.647, -112.194)
  line L10544 (110, -112.284) -> (109.946, -112.366)
  line L10545 (108.519, -112.439) -> (108.423, -112.42)
  line L10546 (110.758, -112.189) -> (110.758, -111.564)
  line L10547 (110.831, -112.366) -> (110.777, -112.284)
  line L10548 (109.946, -112.366) -> (109.864, -112.42)
  line L10549 (110.019, -112.189) -> (110, -112.284)
  line L10550 (108.288, -111.468) -> (108.342, -111.387)
  line L10551 (114.511, -110.985) -> (115.511, -110.985)
  line L10552 (112.508, -111.61) -> (113.211, -111.61)
  line L10553 (108.269, -111.564) -> (108.288, -111.468)
  line L10554 (116.199, -111.932) -> (116.195, -111.926)
  line L10555 (112.435, -111.387) -> (112.489, -111.468)
  line L10556 (112.258, -111.314) -> (112.354, -111.333)
  line L10557 (109.89, -112.888) -> (109.906, -112.816)
  line L10558 (110.216, -112.459) -> (110.354, -112.43)
  line L10559 (108.269, -112.189) -> (108.269, -111.564)
  line L10560 (108.423, -112.42) -> (108.342, -112.366)
  line L10561 (110.913, -112.42) -> (110.912, -112.42)
  line L10562 (109.946, -111.387) -> (110, -111.468)
  line L10563 (110.019, -111.564) -> (110.019, -112.189)
  line L10564 (108.423, -111.333) -> (108.519, -111.314)
  line L10565 (110.75, -112.583) -> (110.913, -112.42)
  line L10566 (108.342, -112.366) -> (108.288, -112.284)
  line L10567 (114.211, -110.985) -> (114.211, -111.135)
  line L10568 (110.831, -111.387) -> (110.912, -111.333)
  line L10569 (116.268, -111.938) -> (116.213, -111.938)
  line L10570 (112.489, -111.468) -> (112.508, -111.564)
  line L10571 (112.354, -111.333) -> (112.435, -111.387)
  line L10572 (110.091, -112.526) -> (110.216, -112.459)
  line L10573 (108.342, -111.387) -> (108.423, -111.333)
  line L10574 (116.195, -111.926) -> (116.193, -111.918)
  line L10575 (110.912, -111.333) -> (111.008, -111.314)
  line L10576 (109.53, -112.439) -> (108.519, -112.439)
  line L10577 (110.031, -112.586) -> (110.091, -112.526)
  line L10578 (116.206, -111.937) -> (116.199, -111.932)
  line L10579 (110.742, -112.575) -> (110.75, -112.583)
  line L10580 (116.213, -111.938) -> (116.206, -111.937)
  line L10581 (115.511, -110.985) -> (115.511, -112.058)
  line L10582 (116.206, -110.75) -> (116.213, -110.748)
  line L10583 (113.211, -111.61) -> (113.211, -110.985)
  line L10584 (108.351, -122.405) -> (108.202, -122.307)
  line L10585 (114.511, -111.135) -> (114.511, -110.985)
  line L10586 (116.193, -110.768) -> (116.195, -110.761)
  line L10587 (109.325, -122.205) -> (109.196, -122.328)
  line L10588 (114.211, -111.535) -> (114.211, -111.935)
  line L10589 (109.487, -121.89) -> (109.424, -122.056)
  line L10590 (116.213, -110.748) -> (116.573, -110.748)
  line L10591 (114.211, -111.935) -> (114.511, -111.935)
  line L10592 (116.195, -110.761) -> (116.199, -110.754)
  line L10593 (109.424, -122.056) -> (109.325, -122.205)
  line L10594 (136.221, -110.487) -> (136.322, -110.471)
  line L10595 (107.929, -121.857) -> (107.912, -121.679)
  line L10596 (114.211, -111.135) -> (114.511, -111.135)
  line L10597 (109.433, -121.345) -> (109.492, -121.513)
  line L10598 (114.511, -111.535) -> (114.211, -111.535)
  line L10599 (111.008, -111.314) -> (112.258, -111.314)
  line L10600 (107.986, -122.026) -> (107.929, -121.857)
  line L10601 (109.063, -120.972) -> (109.213, -121.067)
  line L10602 (116.573, -110.748) -> (116.581, -110.75)
  line L10603 (108.078, -122.179) -> (107.986, -122.026)
  line L10604 (108.895, -120.912) -> (109.063, -120.972)
  line L10605 (108.518, -122.467) -> (108.351, -122.405)
  line L10606 (110.777, -112.284) -> (110.758, -112.189)
  line L10607 (107.912, -121.679) -> (107.934, -121.502)
  line L10608 (110.912, -112.42) -> (110.831, -112.366)
  line L10609 (108.873, -122.474) -> (108.695, -122.49)
  line L10610 (109.339, -121.194) -> (109.433, -121.345)
  line L10611 (109.492, -121.513) -> (109.512, -121.691)
  line L10612 (114.511, -111.935) -> (114.511, -111.535)
  line L10613 (109.512, -121.691) -> (109.512, -121.713)
  line L10614 (116.199, -110.754) -> (116.206, -110.75)
  line L10615 (116.026, -112.194) -> (116.268, -111.952)
  line L10616 (109.196, -122.328) -> (109.042, -122.419)
  line L10617 (109.042, -122.419) -> (108.873, -122.474)
  line L10618 (108.695, -122.49) -> (108.518, -122.467)
  line L10619 (136.557, -111.195) -> (136.445, -111.251)
  line L10620 (136.702, -110.995) -> (136.645, -111.106)
  line L10621 (136.101, -110.424) -> (136.134, -110.428)
  line L10622 (112.508, -111.564) -> (112.508, -111.61)
  line L10623 (109.213, -121.067) -> (109.339, -121.194)
  line L10624 (109.512, -121.713) -> (109.487, -121.89)
  line L10625 (108.371, -120.967) -> (108.54, -120.909)
  line L10626 (136.155, -110.437) -> (136.181, -110.458)
  line L10627 (136.645, -111.106) -> (136.557, -111.195)
  line L10628 (108.202, -122.307) -> (108.078, -122.179)
  line L10629 (136.445, -111.251) -> (136.322, -111.271)
  line L10630 (138.447, -108.799) -> (138.45, -108.777)
  line L10631 (138.45, -108.772) -> (138.451, -108.769)
  line L10632 (143.245, -106.809) -> (143.652, -106.402)
  line L10633 (107.934, -121.502) -> (107.995, -121.335)
  line L10634 (138.392, -110.029) -> (138.384, -110.027)
  line L10635 (136.445, -110.491) -> (136.557, -110.547)
  line L10636 (136.134, -110.428) -> (136.144, -110.434)
  line L10637 (138.374, -110.016) -> (138.372, -110.009)
  line L10638 (138.384, -108.84) -> (138.392, -108.839)
  line L10639 (138.392, -108.839) -> (138.447, -108.839)
  line L10640 (136.702, -110.747) -> (136.722, -110.871)
  line L10641 (138.484, -108.71) -> (140.348, -106.846)
  line L10642 (136.322, -110.471) -> (136.445, -110.491)
  line L10643 (140.348, -106.846) -> (140.366, -106.832)
  line L10644 (138.469, -108.737) -> (138.484, -108.71)
  line L10645 (138.447, -108.839) -> (138.447, -108.799)
  line L10646 (108.718, -120.891) -> (108.895, -120.912)
  line L10647 (138.384, -110.027) -> (138.378, -110.023)
  line L10648 (140.407, -106.818) -> (140.437, -106.809)
  line L10649 (140.437, -106.809) -> (143.245, -106.809)
  line L10650 (138.452, -108.763) -> (138.469, -108.737)
  line L10651 (138.378, -108.845) -> (138.384, -108.84)
  line L10652 (138.77, -110.016) -> (138.766, -110.023)
  line L10653 (140.372, -106.828) -> (140.377, -106.824)
  line L10654 (138.772, -110.009) -> (138.77, -110.016)
  line L10655 (136.198, -111.251) -> (136.087, -111.195)
  line L10656 (107.995, -121.335) -> (108.092, -121.185)
  line L10657 (136.209, -110.476) -> (136.221, -110.487)
  line L10658 (136.645, -110.636) -> (136.702, -110.747)
  line L10659 (108.219, -121.06) -> (108.371, -120.967)
  line L10660 (138.45, -108.777) -> (138.45, -108.772)
  line L10661 (138.752, -110.029) -> (138.392, -110.029)
  line L10662 (138.378, -110.023) -> (138.374, -110.016)
  line L10663 (138.374, -108.851) -> (138.378, -108.845)
  line L10664 (138.772, -108.859) -> (138.772, -110.009)
  line L10665 (136.322, -111.271) -> (136.198, -111.251)
  line L10666 (136.722, -110.871) -> (136.702, -110.995)
  line L10667 (108.092, -121.185) -> (108.219, -121.06)
  line L10668 (140.366, -106.832) -> (140.369, -106.829)
  line L10669 (138.766, -110.023) -> (138.76, -110.027)
  line L10670 (136.557, -110.547) -> (136.645, -110.636)
  line L10671 (136.144, -110.434) -> (136.155, -110.437)
  line L10672 (136.181, -110.458) -> (136.209, -110.476)
  line L10673 (108.54, -120.909) -> (108.718, -120.891)
  line L10674 (140.369, -106.829) -> (140.372, -106.828)
  line L10675 (140.377, -106.824) -> (140.407, -106.818)
  line L10676 (138.451, -108.769) -> (138.452, -108.763)
  line L10677 (138.372, -110.009) -> (138.372, -108.859)
  line L10678 (122.769, -114.159) -> (115.66, -114.159)
  line L10679 (114.891, -113.646) -> (114.834, -113.535)
  line L10680 (115.214, -113.011) -> (115.338, -113.031)
  line L10681 (115.45, -113.087) -> (115.538, -113.176)
  line L10682 (122.802, -114.151) -> (122.769, -114.159)
  line L10683 (115.091, -113.031) -> (115.214, -113.011)
  line L10684 (114.834, -113.535) -> (114.814, -113.411)
  line L10685 (119.55, -112.335) -> (119.55, -112.485)
  line L10686 (119.55, -112.485) -> (118.55, -112.485)
  line L10687 (115.594, -114.148) -> (115.585, -114.141)
  line L10688 (115.538, -113.176) -> (115.595, -113.287)
  line L10689 (114.979, -113.087) -> (115.091, -113.031)
  line L10690 (115.66, -114.159) -> (115.628, -114.151)
  line L10691 (122.442, -112.439) -> (121.93, -112.439)
  line L10692 (115.091, -113.791) -> (114.979, -113.735)
  line L10693 (115.574, -114.139) -> (115.547, -114.118)
  line L10694 (115.595, -113.535) -> (115.569, -113.585)
  line L10695 (122.845, -114.142) -> (122.835, -114.148)
  line L10696 (118.536, -112.421) -> (118.533, -112.424)
  line L10697 (115.338, -113.031) -> (115.45, -113.087)
  line L10698 (114.814, -113.411) -> (114.834, -113.287)
  line L10699 (115.628, -114.151) -> (115.594, -114.148)
  line L10700 (115.614, -113.411) -> (115.595, -113.535)
  line L10701 (115.519, -114.1) -> (115.228, -113.809)
  line L10702 (122.835, -114.148) -> (122.802, -114.151)
  line L10703 (121.753, -112.366) -> (121.699, -112.284)
  line L10704 (115.585, -114.141) -> (115.574, -114.139)
  line L10705 (115.547, -114.118) -> (115.519, -114.1)
  line L10706 (122.45, -112.463) -> (122.449, -112.46)
  line L10707 (122.856, -114.139) -> (122.845, -114.142)
  line L10708 (115.214, -113.811) -> (115.091, -113.791)
  line L10709 (118.55, -112.485) -> (118.55, -112.41)
  line L10710 (118.533, -112.424) -> (118.53, -112.425)
  line L10711 (138.372, -108.859) -> (138.374, -108.851)
  line L10712 (114.891, -113.176) -> (114.979, -113.087)
  line L10713 (114.979, -113.735) -> (114.891, -113.646)
  line L10714 (114.834, -113.287) -> (114.891, -113.176)
  line L10715 (121.834, -112.42) -> (121.753, -112.366)
  line L10716 (121.68, -112.189) -> (121.68, -111.86)
  line L10717 (115.595, -113.287) -> (115.614, -113.411)
  line L10718 (123.109, -113.1) -> (123.08, -113.084)
  line L10719 (138.76, -110.027) -> (138.752, -110.029)
  line L10720 (122.882, -114.118) -> (122.856, -114.139)
  line L10721 (115.228, -113.809) -> (115.214, -113.811)
  line L10722 (115.569, -113.585) -> (115.743, -113.759)
  line L10723 (123.113, -113.101) -> (123.111, -113.101)